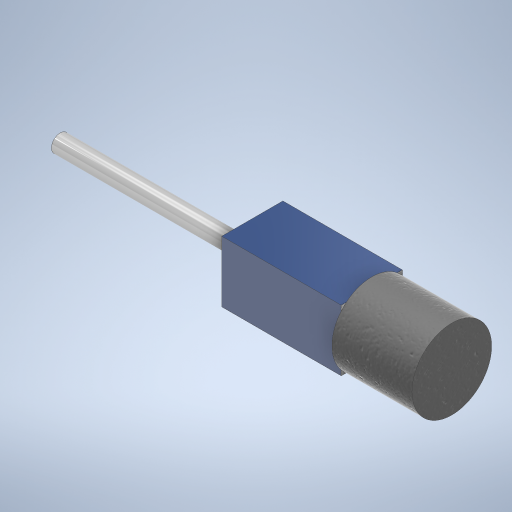
# Autodesk Inventor part: MotorAxel
Saved by Autodesk Inventor 2023 (Build 270158000, 158)
## iProperties
Created: 2022-08-31
Part Number: MotorAxel
Material: Generic
Document SubType Name: Modeling
Designer: PC
Density: 1 g/cm^3
Appearance: Aluminum Cast
Author: PC
Autodesk Inventor part; units mm, degrees
ref_plane "YZ Plane" through (0, 0, 0) normal (1, 0, 0) x (0, 1, 0)
ref_plane "XZ Plane" through (0, 0, 0) normal (0, 1, 0) x (-1, 0, 0)
ref_plane "XY Plane" through (0, 0, 0) normal (0, 0, 1) x (1, 0, 0)
sketch "Sketch1" plane through (0, 0, 0) normal (1, 0, 0) x (0, 1, 0)
  line L0 (22.225, 22.225) -> (-22.225, 22.225)
  line L1 (-22.225, 22.225) -> (-22.225, -22.225)
  line L2 (-22.225, -22.225) -> (22.225, -22.225)
  line L3 (22.225, -22.225) -> (22.225, 22.225)
  line L4 (22.225, 22.225) -> (-22.225, -22.225) construction
  line L5 (-22.225, 22.225) -> (22.225, -22.225) construction
  point P0 (0, 0)
  dimension "d0" = 44.45
  dimension "d1" = 44.45
  constraints: 12 end point, 2 midpoint, 2 parallel, 1 horizontal, 1 perpendicular
  measures "d0" distance of L1.end L2.end
  measures "d1" distance of L0.end L1.end
extrude "Extrusion1" add sketch "Sketch1" along normal blind 86.868
sketch "Sketch2" plane through (86.868, 0, 0) normal (1, 0, 0) x (0, 0, -1)
  circle A0 centre (0, 0) radius 28.956
  dimension "d4" = 57.912
  constraints: 1 centre point, 1 coincident
  measures "d4" diameter of A0
extrude "Extrusion2" add sketch "Sketch2" along normal blind 58.166
sketch "Sketch3" plane through (0, 0, 0) normal (-1, 0, 0) x (0, 0, 1)
  circle A0 centre (0, 0) radius 6.35
  dimension "d7" = 12.7
  constraints: 1 centre point, 1 coincident
  measures "d7" diameter of A0
extrude "Extrusion3" add sketch "Sketch3" along normal blind 139.7
equation "\"d1\" = d0"
body "Solid1"
